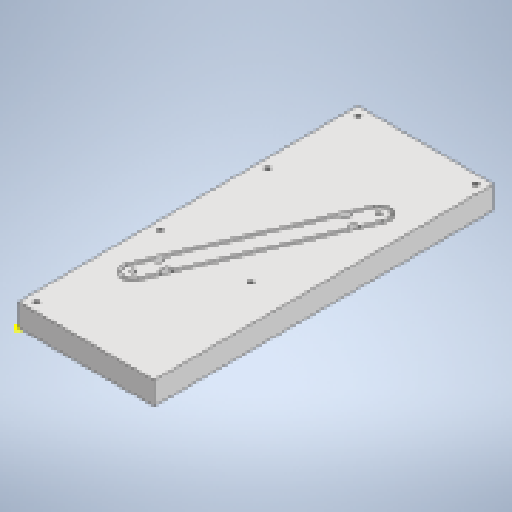
# Autodesk Inventor part: FlexK7Holder
Saved by Autodesk Inventor 2023 (Build 270158000, 158)
## iProperties
Created: 2023-03-30
Part Number: FlexK7Holder
Material: Generic
Document SubType Name: Modeling
Designer: Nathann
Density: 1 g/cm^3
Appearance: Default
Author: Nathann
Autodesk Inventor part; units mm, degrees
ref_plane "YZ Plane" through (0, 0, 0) normal (1, 0, 0) x (0, 1, 0)
ref_plane "XZ Plane" through (0, 0, 0) normal (0, 1, 0) x (-1, 0, 0)
ref_plane "XY Plane" through (0, 0, 0) normal (0, 0, 1) x (1, 0, 0)
sketch "Sketch1" plane through (0, 0, 0) normal (0, 1, 0) x (-1, 0, 0)
  line L0 (0, 0) -> (-60, 0)
  line L1 (-60, 0) -> (-60, -150)
  line L2 (-60, -150) -> (0, -150)
  line L3 (0, -150) -> (0, 0)
  dimension "d0" = 150
  dimension "d1" = 60
  constraints: 8 end point, 2 parallel, 1 horizontal, 1 perpendicular
  measures "d0" distance of L0.end L1.end
  measures "d1" distance of L0.start L0.end
extrude "Extrusion1" add sketch "Sketch1" along normal blind 10
sketch "Sketch2" plane through (0, 0, 0) normal (0, -1, 0) x (1, 0, 0)
  circle A0 centre (4, -146) radius 1.325 projected
  circle A1 centre (56, -146) radius 1.325 projected
  circle A2 centre (4, -4) radius 1.325 projected
  circle A3 centre (4, -58.741) radius 1.325 projected
  circle A4 centre (44, -58.741) radius 1.325 projected
  circle A5 centre (4, -106.0864) radius 1.325 projected
  point P0 (0, 0)
sketch "Sketch3" plane through (0, 0, 0) normal (0, -1, 0) x (1, 0, 0)
  circle A0 centre (4, -146) radius 1.325 projected
  circle A1 centre (4, -146) radius 1.1
  circle A2 centre (56, -146) radius 1.325 projected
  circle A3 centre (56, -146) radius 1.1
  circle A4 centre (4, -106.0864) radius 1.1
  circle A5 centre (4, -58.741) radius 1.1
  circle A6 centre (44, -58.741) radius 1.1
  circle A7 centre (4, -4) radius 1.1
  point P0 (0, 0)
  dimension "d4" = 2.2
  dimension "d5" = 2.2
  dimension "d6" = 2.2
  dimension "d7" = 2.2
  dimension "d8" = 2.2
  dimension "d9" = 2.2
  constraints: 6 centre point, 6 coincident
  measures "d4" diameter of A1
  measures "d5" diameter of A3
  measures "d6" diameter of A4
  measures "d7" diameter of A6
  measures "d8" diameter of A5
  measures "d9" diameter of A7
extrude "Extrusion2" cut sketch "Sketch3" against normal blind 10 contours A1 | A3 | A4 | A5 | A6 | A7
thread "Thread1" size "M2.5x0.45" class "6H" standard "ANSI Metric M Profile" length 10
thread "Thread2" size "M2.5x0.45" class "6H" standard "ANSI Metric M Profile" length 10
thread "Thread3" size "M2.5x0.45" class "6H" standard "ANSI Metric M Profile" length 10
thread "Thread4" size "M2.5x0.45" class "6H" standard "ANSI Metric M Profile" length 10
thread "Thread5" size "M2.5x0.45" class "6H" standard "ANSI Metric M Profile" length 10
thread "Thread6" size "M2.5x0.45" class "6H" standard "ANSI Metric M Profile" length 10
sketch "Sketch4" plane through (0, 10, 0) normal (0, 1, 0) x (1, 0, 0)
  circle A0 centre (13.8775, 36.8056) radius 1.1
  circle A1 centre (46.1225, 113.1944) radius 1.1
  arc A2 (36.6332, 8.5) -> (15.5373, 47.236) centre (30, 30) ccw projected
  arc A3 (30.5692, 97.5072) -> (51.5, 113.3668) centre (30, 120) ccw projected
  arc A4 (36.6332, 8.5) -> (15.5373, 47.236) centre (30, 30) ccw projected
  line L0 (9.2711, 38.75) -> (41.5161, 115.1389)
  line L1 (18.4839, 34.8611) -> (50.7289, 111.25)
  arc A5 (9.2711, 38.75) -> (18.4839, 34.8611) centre (13.8775, 36.8056) ccw
  arc A6 (50.7289, 111.25) -> (41.5161, 115.1389) centre (46.1225, 113.1944) ccw
  line L2 (30, 30) -> (22.4986, 30)
  line L3 (30, 120) -> (36.6332, 120)
  line L4 (41.5161, 115.1389) -> (50.7289, 111.25)
  line L5 (9.2711, 38.75) -> (18.4839, 34.8611)
  line L6 (30, 30) -> (13.8775, 36.8056)
  line L7 (46.1225, 113.1944) -> (30, 120)
  line L8 (13.8775, 36.8056) -> (46.1225, 113.1944)
  circle A7 centre (30, 30) radius 17.5
  circle A8 centre (30, 120) radius 17.5
  circle A9 centre (13.8775, 36.8056) radius 3.5
  circle A10 centre (46.1225, 113.1944) radius 3.5
  line L9 (10.653, 38.1667) -> (42.898, 114.5556)
  line L10 (49.347, 111.8333) -> (17.102, 35.4444)
  circle A11 centre (14.5419, 47.3795) radius 2
  line L11 (14.5419, 47.3795) -> (20.9909, 44.6573)
  circle A12 centre (20.9909, 44.6573) radius 2
  circle A13 centre (39.0091, 105.3427) radius 2
  circle A14 centre (45.4581, 102.6205) radius 2
  line L12 (39.0091, 105.3427) -> (45.4581, 102.6205)
  point P0 (0, 0)
  point P1 (45.6947, 112.181)
  point P2 (45.6631, 112.195)
  point P3 (44.4457, 110.1222)
  point P4 (44.7614, 109.9699)
  point P5 (13.7641, 45.5369)
  point P6 (15.3197, 49.2221)
  point P7 (38.2313, 103.5001)
  point P8 (39.7869, 107.1853)
  point P9 (46.2359, 104.4631)
  point P10 (44.6803, 100.7779)
  point P11 (21.7687, 46.4999)
  point P12 (20.2131, 42.8147)
  point P13 (38.1416, 107.1448)
  point P14 (37.4074, 104.145)
  point P15 (36.7532, 103.8555)
  point P16 (40.801, 106.2309)
  point P17 (37.1127, 104.7073)
  point P18 (47.3889, 118.0314)
  point P19 (22.8873, 45.2927)
  point P20 (22.5926, 45.855)
  point P21 (23.2468, 46.1445)
  point P22 (47.1543, 116.5389)
  dimension "d27" = 35
  dimension "d24" = 10
  dimension "d25" = 22.5
  dimension "d26" = 35
  dimension "d28" = 7
  dimension "d29" = 7
  dimension "d30" = 4
  dimension "d31" = 4
  dimension "d32" = 90
  dimension "d33" = 4
  dimension "d34" = 4
  dimension "d35" = 10
  dimension "d36" = 10
  dimension "d39" = 2.2
  dimension "d40" = 2.2
  constraints: 26 end point, 11 centre point, 10 point on circle, 9 point on line, 6 coincident, 4 perpendicular, 4 tangent, 2 horizontal, 2 midpoint, 1 parallel, 3 other
  measures "d24" distance between parallel lines of L0 L1
  measures "d25" radius of A2
  measures "d26" diameter of A7
  measures "d28" diameter of A9
  measures "d29" diameter of A10
  measures "d30" diameter of A11
  measures "d31" diameter of A12
  measures "d32" angle of L9 L12
  measures "d33" diameter of A13
  measures "d34" diameter of A14
  measures "d35" distance of L10.start L12.end
  measures "d36" distance from line of L11.end L6
  measures "d39" diameter of A0
  measures "d40" diameter of A1
extrude "Extrusion3" cut sketch "Sketch4" against normal blind 10 contours A0 L5 A7 | A7 L8 A0 | A0 A7 L5 | L8 L5 A0 | A7 A0 L5 | L10 A12 L1 L5 | L5 A5 A7 A9 | A12 L11 A7 | A7 L11 L10 A12 | A7 A5 L5 A9 | L10 A7 A12 L1 | L5 L0 A11 L9 | L11 A12 L10 A7 | A7 L10 L11 | A11 L0 L9 | L9 L11 A11 | L11 L9 A11 | L10 A12 A7 | L10 A2 L1 A7 A12 | A12 A7 L1 | L10 A14 L1 A2 | L0 A3 L9 A11 | A14 A3 L12 L10 | L10 A3 A14 L1 | A3 L0 A8 A13 L9 | A14 L12 A3 | L12 A3 L10 | A13 A8 L9 | L9 A8 L12 A13 | L12 A14 L10 A3 | L12 A8 A13 | L0 A13 A8 | A14 A3 L1 | L10 A14 A3 | L9 L12 A8 | A8 A13 L0 L9 | L10 L4 A3 A14 | L8 L4 A1 | A1 A8 L8 | A10 A8 A6 L4 | L12 L9 A13 A8 | A1 L4 A8 | L4 A8 A1 | L4 A1 A8 | L9 A13 L0 L4 | L4 A6 A8 A10
equation "\"d27\" = d26"
equation "\"d31\" = d30"
equation "\"d33\" = d30"
equation "\"d34\" = d30"
body "Solid1"
